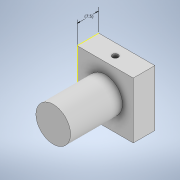
# Autodesk Inventor part: HDzero runcam with micro spacer
Saved by Autodesk Inventor 2020 (Build 240168000, 168)
## iProperties
Created: 2022-05-06
Part Number: HDzero runcam with micro spacer
Material: Generic
Document SubType Name: Modeling
Designer: Steven
Density: 1 g/cm^3
Appearance: Default
Author: Steven
Autodesk Inventor part; units mm, degrees
ref_plane "YZ Plane" through (0, 0, 0) normal (1, 0, 0) x (0, 1, 0)
ref_plane "XZ Plane" through (0, 0, 0) normal (0, 1, 0) x (-1, 0, 0)
ref_plane "XY Plane" through (0, 0, 0) normal (0, 0, 1) x (1, 0, 0)
sketch "Sketch1" plane through (0, 0, 0) normal (0, 0, 1) x (1, 0, 0)
  line L0 (0, 0) -> (19.5, 0)
  line L1 (19.5, 0) -> (19.5, 19.5)
  line L2 (19.5, 19.5) -> (0, 19.5)
  line L3 (0, 19.5) -> (0, 0)
  dimension "d0" = 19.5
  dimension "d1" = 19.5
  constraints: 8 end point, 2 parallel, 1 horizontal, 1 perpendicular
  measures "d0" distance of L2.end L1.end
  measures "d1" distance of L1.end L0.end
extrude "Extrusion1" add sketch "Sketch1" along normal blind 7.5
sketch "Sketch6" plane through (0, 0, 7.5) normal (0, 0, 1) x (1, 0, 0)
  line L0 (19.5, 0) -> (19.5, 19.5) construction
  line L1 (19.5, 9.75) -> (0, 9.75) construction
  line L2 (0, 19.5) -> (0, 0) construction
  circle A0 centre (9.75, 9.75) radius 6
  dimension "d14" = 12
  constraints: 3 midpoint, 2 end point, 1 centre point
  measures "d14" diameter of A0
sketch "Sketch7" plane through (0, 0, 0) normal (-1, 0, 0) x (0, 0, 1)
  line L0 (0, 19.5) -> (0, 0) projected
  line L1 (0, 0) -> (7.5, 0) projected
  line L2 (7.5, 19.5) -> (7.5, 0) projected
  line L3 (0, 19.5) -> (7.5, 19.5) projected
  dimension "d15" = 7.5
  measures "d15" distance of L0.start L2.start
extrude "Extrusion4" add sketch "Sketch6" along normal blind 18
sketch "Sketch8" plane through (0, 19.5, 0) normal (0, 1, 0) x (1, 0, 0)
  line L0 (19.5, 0) -> (0, 0) projected
  line L1 (0, 0) -> (19.5, 0) construction
  line L2 (9.75, 0) -> (9.75, -5) construction
  line L3 (9.75, -5) -> (11.9374, -5) construction
  circle A0 centre (9.75, -4) radius 1
  dimension "d18" = 5
  dimension "d19" = 2
  constraints: 4 end point, 1 centre point, 1 horizontal, 1 midpoint, 1 point on line, 1 tangent, 1 vertical
  measures "d18" distance of L2.start L2.end
  measures "d19" diameter of A0
extrude "Extrusion5" cut sketch "Sketch8" against normal up to surface (19.5 mm away)
body "Solid1"
